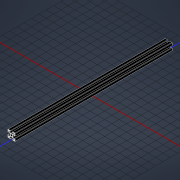
# Autodesk Inventor part: Extrusion_20x20x430
Saved by Autodesk Inventor 2022 (Build 260153000, 153)
## iProperties
Created: 2022-03-06
Part Number: Extrusion_20x20x430
Material: Aluminium 6061
Document SubType Name: Modeling
Designer: sleib
Density: 2.7 g/cm^3
Appearance: Eloxiert - Schwarz
Author: sleib
Autodesk Inventor part; units mm, degrees
ref_plane "YZ Plane" through (0, 0, 0) normal (1, 0, 0) x (0, 1, 0)
ref_plane "XZ Plane" through (0, 0, 0) normal (0, 1, 0) x (-1, 0, 0)
ref_plane "XY Plane" through (0, 0, 0) normal (0, 0, 1) x (1, 0, 0)
sketch "Skizze1" plane through (0, 0, 0) normal (0, 0, 1) x (1, 0, 0)
  line L0 (3.7, 0) -> (4, 0.5196)
  line L1 (4, 0.5196) -> (4, 2.9393)
  line L2 (4, 2.9393) -> (7.0607, 6)
  line L3 (7.0607, 6) -> (8, 6)
  line L4 (8, 6) -> (8, 3)
  line L5 (8, 3) -> (10, 3)
  line L6 (10, 3) -> (10, 9)
  arc A0 (10, 9) -> (9, 10) centre (9, 9) ccw
  line L7 (9, 10) -> (3, 10)
  line L8 (3, 10) -> (3, 8)
  line L9 (3, 8) -> (6, 8)
  line L10 (6, 8) -> (6, 7.0607)
  line L11 (6, 7.0607) -> (2.9393, 4)
  line L12 (2.9393, 4) -> (0.5196, 4)
  line L13 (0.5196, 4) -> (0, 3.7)
  circle A1 centre (0, 0) radius 2.56
  line L14 (0, 0) -> (9.7071, 9.7071) construction
  line L15 (-14.2899, 0) -> (14.2899, 0) construction
  line L16 (0, -14.2899) -> (0, 14.2899) construction
  line L17 (0, 3.7) -> (-0.5196, 4)
  line L18 (-0.5196, 4) -> (-2.9393, 4)
  line L19 (-3, 8) -> (-3, 10)
  line L20 (-4, 0.5196) -> (-3.7, 0)
  line L21 (-4, 2.9393) -> (-4, 0.5196)
  line L22 (-6, 7.0607) -> (-6, 8)
  line L23 (-6, 8) -> (-3, 8)
  line L24 (-7.0607, 6) -> (-4, 2.9393)
  line L25 (0, 0) -> (-9.7071, 9.7071) construction
  line L26 (-8, 6) -> (-7.0607, 6)
  line L27 (-2.9393, 4) -> (-6, 7.0607)
  line L28 (-8, 3) -> (-8, 6)
  line L29 (-10, 3) -> (-8, 3)
  arc A2 (-9, 10) -> (-10, 9) centre (-9, 9) ccw
  line L30 (-10, 9) -> (-10, 3)
  line L31 (-3, 10) -> (-9, 10)
  line L32 (-3.7, 0) -> (-4, -0.5196)
  line L33 (-4, -0.5196) -> (-4, -2.9393)
  line L34 (-8, -3) -> (-10, -3)
  line L35 (-0.5196, -4) -> (0, -3.7)
  line L36 (-2.9393, -4) -> (-0.5196, -4)
  line L37 (-7.0607, -6) -> (-8, -6)
  line L38 (-8, -6) -> (-8, -3)
  line L39 (-6, -7.0607) -> (-2.9393, -4)
  line L40 (0, 0) -> (-9.7071, -9.7071) construction
  line L41 (-6, -8) -> (-6, -7.0607)
  line L42 (-4, -2.9393) -> (-7.0607, -6)
  line L43 (-3, -8) -> (-6, -8)
  line L44 (-3, -10) -> (-3, -8)
  arc A3 (-10, -9) -> (-9, -10) centre (-9, -9) ccw
  line L45 (-9, -10) -> (-3, -10)
  line L46 (-10, -3) -> (-10, -9)
  line L47 (0, -3.7) -> (0.5196, -4)
  line L48 (0.5196, -4) -> (2.9393, -4)
  line L49 (3, -8) -> (3, -10)
  line L50 (4, -0.5196) -> (3.7, 0)
  line L51 (4, -2.9393) -> (4, -0.5196)
  line L52 (6, -7.0607) -> (6, -8)
  line L53 (6, -8) -> (3, -8)
  line L54 (7.0607, -6) -> (4, -2.9393)
  line L55 (0, 0) -> (9.7071, -9.7071) construction
  line L56 (8, -6) -> (7.0607, -6)
  line L57 (2.9393, -4) -> (6, -7.0607)
  line L58 (8, -3) -> (8, -6)
  line L59 (10, -3) -> (8, -3)
  arc A4 (9, -10) -> (10, -9) centre (9, -9) ccw
  line L60 (10, -9) -> (10, -3)
  line L61 (3, -10) -> (9, -10)
  point P0 (-3.7, 0)
  point P1 (0, -3.7)
  dimension "d14" = 1.5
  dimension "d15" = 3
  dimension "d16" = 4
  dimension "d17" = 0.3
  dimension "d18" = 2
  dimension "d19" = 6
  dimension "d20" = 10
  dimension "d21" = 10
  dimension "d22" = 2
  dimension "d23" = 3
  dimension "d24" = 6
  dimension "d25" = 1
  dimension "d26" = 4
  dimension "d27" = 0.3
  dimension "d28" = 0.5196
  dimension "d29" = 0.5196
  dimension "d30" = 5.12
  dimension "d33" = 360
  constraints: 120 end point, 9 point on circle, 6 coincident, 6 perpendicular, 6 point on line, 5 centre point, 2 tangent, 1 midpoint, 144 other
  measures "d14" distance between parallel lines of L2 L11
  measures "d15" distance between parallel lines of L5 L15
  measures "d16" distance between parallel lines of L4 L1
  measures "d17" distance from line of L0.start L1
  measures "d18" distance between parallel lines of L6 L4
  measures "d19" distance between parallel lines of L15 L3
  measures "d20" distance between parallel lines of L6 L16
  measures "d21" distance between parallel lines of L15 L7
  measures "d22" distance between parallel lines of L9 L7
  measures "d23" distance between parallel lines of L8 L16
  measures "d24" distance between parallel lines of L10 L16
  measures "d25" radius of A0
  measures "d26" distance between parallel lines of L12 L9
  measures "d27" distance from line of L12 L13.end
  measures "d28" horizontal distance of L13.start L13.end
  measures "d29" vertical distance of L0.start L1.start
  measures "d30" diameter of A1
extrude "Extrusion1" add sketch "Skizze1" along normal mid plane 430
